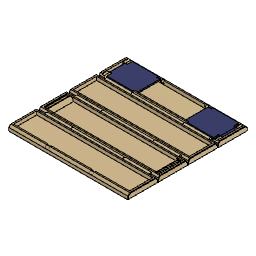
RollupBoard (Autodesk Fusion 360 design; units mm, degrees)
Autodesk Fusion 360 part; units mm, degrees
note: some values were not read from the file. Chosen so that the rebuilt part matches the saved one: a side; which face or edge a step refers to. Set by a fixed rule: which sketch regions a step uses.
sketch "Sketch3" plane through (0, 0, 0) normal (1, 0, 0) x (0, 1, 0)
  line L0 (0.25, 0) -> (45.75, 0)
  line L1 (46, 0) -> (46, 8) construction
  circle A0 centre (46, 5) radius 0.875 construction
  line L2 (38.0198, 12.9802) -> (46, 5) construction
  circle A1 centre (46, 5) radius 1.225
  arc A2 (47.8562, 3.1438) -> (43.9755, 6.6709) centre (46, 5) ccw
  line L3 (47.8562, 3.1438) -> (45.75, 1.0377)
  line L4 (2.9898, 47.3471) -> (2.9889, 8.0542) construction
  line L5 (-5, 5.25) -> (-5, 50.75) construction
  line L6 (43, 8.3536) -> (43, 9.3938) construction
  line L7 (51, 50.75) -> (51, 5.25) construction
  line L8 (24.7755, 27.5722) -> (42.5, 27.5722) construction
  line L9 (42.5, 27.5722) -> (42.5, 9.8477) construction
  line L10 (42.5, 9.8477) -> (24.7755, 9.8477) construction
  line L11 (24.7755, 9.8477) -> (24.7755, 27.5722) construction
  circle A3 centre (13.4891, 17.5722) radius 10 construction
  line L12 (24.7755, 9.8477) -> (42.5, 27.5722) construction
  line L13 (46, 8) -> (42.6464, 8) construction
  line L14 (40.6464, 2.5) -> (40.6464, 8)
  line L15 (3, 10.1318) -> (-3.0001, 10.1756) construction
  line L16 (-3.0001, 45.4688) -> (3, 45.425) construction
  line L17 (-3.0001, 10.1756) -> (-3.0001, 45.4688) construction
  line L18 (48.5, 10.3536) -> (43, 10.3536) construction
  line L19 (49.0395, 45.534) -> (48.5, 10.3536) construction
  line L20 (43.0002, 45.5096) -> (49.0395, 45.534) construction
  circle A4 centre (13.4891, 38.0722) radius 10 construction
  line L21 (-3.0001, 27.8222) -> (-12.3549, 27.8222) construction
  line L22 (5.453, 47.7007) -> (5.4663, 53.6839) construction
  line L23 (5.4663, 53.6839) -> (40.6464, 53.1444) construction
  line L24 (42.6464, 47.6444) -> (41.608, 47.6437) construction
  line L25 (0.25, 55.6444) -> (45.75, 55.6444) construction
  line L26 (40.6464, 53.1444) -> (40.6464, 47.6444) construction
  line L27 (24.7755, 28.0722) -> (42.5, 28.0722) construction
  line L28 (24.7755, 45.7968) -> (24.7755, 28.0722) construction
  line L29 (42.5, 28.0722) -> (42.5, 45.7968) construction
  line L30 (42.5, 45.7968) -> (24.7755, 45.7968) construction
  line L31 (23, 0) -> (23, 6.2006) construction
  line L32 (45.75, 4.8964) -> (42.6464, 8)
  line L33 (45.75, 4.8964) -> (45.75, 0)
  line L34 (44.1438, 3.1438) -> (46.25, 1.0377) construction
  arc A5 (43.9755, 6.6709) -> (44.1438, 3.1438) centre (46, 5) ccw construction
  arc A6 (43.727, 6.9194) -> (43.8964, 2.8964) centre (46, 5) ccw
  line L35 (43.8964, 2.8964) -> (45.75, 1.0427)
  line L36 (2.1036, 2.8964) -> (0.25, 1.0427)
  arc A7 (2.1036, 2.8964) -> (2.273, 6.9194) centre (0, 5) ccw
  line L37 (0.25, 4.8964) -> (3.3536, 8)
  arc A8 (2.0245, 6.6709) -> (-1.8562, 3.1438) centre (0, 5) ccw
  circle A9 centre (0, 5) radius 0.875 construction
  line L38 (-1.8562, 3.1438) -> (0.25, 1.0377)
  line L39 (0.25, 4.8964) -> (0.25, 0)
  line L40 (42.6464, 8) -> (3.3536, 8)
  line L41 (5.3536, 2.5) -> (5.3536, 8)
  line L42 (5.3536, 2.5) -> (40.6464, 2.5)
  circle A10 centre (0, 5) radius 1.225
  circle A11 centre (46, 5) radius 1.115
  point P0 (33.6377, 18.7099)
  dimension "d10" = 46
  dimension "d11" = 1.75
  dimension "d15" = 5
  dimension "d16" = 45
  dimension "d17" = 0.35
  dimension "d18" = 1.75
  dimension "d25" = 17.7245
  dimension "d28" = 20
  dimension "d37" = 20.5
  dimension "d38" = 0.5
  dimension "d39" = 0.5
  dimension "d40" = 10.5
  dimension "d41" = 23
  dimension "d56" = 0.25
  dimension "d57" = 0.25
  dimension "d58" = 45
  dimension "d59" = 0.35
  dimension "d60" = 0.25
  dimension "d61" = 8
  dimension "d62" = 2
  dimension "d63" = 2.5
  dimension "d65" = 0.35
  dimension "d78" = 0.24
  constraint horizontal L0
  constraint vertical L1
  constraint coincident L1 A0.centre
  constraint coincident A0.centre L2.end
  constraint concentric A0 A1
  constraint tangent A2 L3
  constraint coincident L1.start L0
  constraint symmetric L0.end L2 L7.end
  constraint symmetric L13.end L2 L6.start
  constraint symmetric L2 L0.start L7.start
  constraint horizontal L8
  constraint vertical L9
  constraint horizontal L10
  constraint vertical L11
  constraint equal L10 L11
  constraint midpoint L12 P0
  constraint symmetric L2 L14.start L18.start
  constraint symmetric L2 L14.end L18.end
  constraint equal A3 A4
  constraint midpoint L17 L21.start
  constraint perpendicular L17 L21
  constraint symmetric A3.centre A4.centre L21
  constraint symmetric L0.end L21 L25.end
  constraint symmetric L13.end L21 L24.start
  constraint symmetric L0.start L21 L25.start
  constraint symmetric L14.start L21 L23.end
  constraint symmetric L14.end L21 L26.end
  constraint symmetric L8.start L21 L27.start
  constraint symmetric L8.end L21 L27.end
  constraint symmetric L9.end L21 L29.end
  constraint symmetric L10.end L21 L28.start
  constraint perpendicular L0 L31
  constraint coincident L0 L31.start
  constraint parallel L2 L32
  constraint coincident L13.end L32.end
  constraint coincident L32 A2.end
  constraint parallel L1 L33
  constraint coincident L33 L3.end
  constraint symmetric L1 A2.start L34.start
  constraint symmetric L1 L3.end L34.end
  constraint coincident A2.end A5.start
  constraint coincident L32 A6.start
  constraint parallel L34 L35
  constraint coincident A6.end L35.start
  constraint tangent A6 L35
  constraint coincident L33 L35.end
  constraint coincident L0.end L33.end
  constraint coincident origin L0
  constraint vertical L14
  constraint symmetric A0 L31 A9
  constraint symmetric A2.start L31 A8.end
  constraint symmetric A2 L31 A8
  constraint symmetric L32.start L31 L37.start
  constraint symmetric L31 L13.end L37.end
  constraint symmetric L31 A2.end A8.start
  constraint symmetric L31 L0.end L0.start
  constraint symmetric L31 L3.end L38.end
  constraint symmetric L31 A6.start A7.end
  constraint symmetric L31 A6.end L36.start
  constraint symmetric L31 A6 A7
  constraint symmetric L31 L35.end L36.end
  constraint horizontal L40
  constraint coincident L37.end L40.end
  constraint horizontal L13
  constraint coincident L14.end L40
  constraint symmetric L14.start L31 L41.start
  constraint symmetric L14.end L31 L41.end
  constraint concentric A7 A10
  constraint concentric A2 A11
  measures "d10" distance of origin L1.start
  measures "d11" diameter of A0
  measures "d15" distance of L1.start A0.centre
  measures "d16" angle of L1 L2
  measures "d17" distance of A0 A1
  measures "d18" distance of A0 A2
  measures "d25" distance of L8.start L8.end
  measures "d28" diameter of A3
  measures "d37" distance of A3.centre A4.centre
  measures "d38" distance of L8 L27
  measures "d39" distance of L6 L9
  measures "d40" distance of L4 A3.centre
  measures "d41" distance of origin L31.start
  measures "d56" distance of L2 L32
  measures "d57" distance of L1 L33
  measures "d58" angle of L1 L3
  measures "d59" distance of A5 A6
  measures "d60" distance of origin L0.start
  measures "d61" distance of L1.start L1.end
  measures "d62" distance of L13.end L14.end
  measures "d63" distance of L0 L14.start
  measures "d65" distance of A9 A10
  measures "d78" distance of A0 A11
extrude "Extrude2" add sketch "Sketch3" along normal mid plane 184 contours L0 L14 L32 L33 A6 L35 L36 A7 L37 L39 L40 L41 L42 | L36 A7 L37 L39 A10 | A1 L32 L33 A6 L35 | L14 L40 L41 L42 makes body 1
extrude "Extrude3" cut sketch "Sketch3" along normal up to surface (89 mm away) and the other way up to surface (89 mm away) contours L14 L40 L41 L42 bodies 1
extrude "Extrude8" add sketch "Sketch3" along normal blind 40 from surface at 40 contours A1 A2 L3 L32 L33 | A1 L32 L33 A11 | A1 L32 L33 A11 bodies 1
mirror "Mirror3" about plane through (0, 0, 0) normal (1, 0, 0) of "Extrude8"
extrude "Extrude9" cut sketch "Sketch3" along normal up to surface (80 mm away) from surface at -40 contours A1 L32 L33 A6 L35 bodies 1
extrude "Extrude10" add sketch "Sketch3" along normal mid plane 79.3 contours L37 A8 L38 L39 A10 bodies 1
extrude "Extrude11" cut sketch "Sketch3" along normal blind 40.7 from surface at 39.65 contours L36 A7 L37 L39 A10 bodies 1
mirror "Mirror4" about plane through (0, 0, 0) normal (1, 0, 0) of "Extrude11"
copy_body "CopyPasteBodies4" bodies 1 makes body 2
move_body "Move4" bodies 2 to x (1, 0, 0) y (0, 1, 0) z (0, 0, 1) at (0, 46, 0)
extrude "Extrude12" add sketch "Sketch3" along normal mid plane 184 separate body contours L0 L14 L32 L33 A6 L35 L36 A7 L37 L39 L40 L41 L42 | L36 A7 L37 L39 A10 | A1 L32 L33 A6 L35 | L37 L39 A10 | L14 L40 L41 L42 picked at (0.8957, 5.0245) makes body 3
extrude "Extrude13" cut sketch "Sketch3" along normal up to surface (89 mm away) and the other way up to surface (89 mm away) contours L14 L40 L41 L42 bodies 3
extrude "Extrude14" add sketch "Sketch3" along normal blind 40 from surface at 40 contours A1 A2 L3 L32 L33 | A1 L32 L33 A11 | A1 L32 L33 A11 bodies 3
mirror "Mirror5" about plane through (0, 0, 0) normal (1, 0, 0) of "Extrude14"
extrude "Extrude15" cut sketch "Sketch3" along normal up to surface (80 mm away) from surface at -40 contours A1 L32 L33 A6 L35 bodies 3
move_body "Move6" bodies 3 to x (1, 0, 0) y (0, 1, 0) z (0, 0, 1) at (0, -46, 0)
extrude "Extrude16" add sketch "Sketch3" along normal mid plane 184 separate body contours L0 L14 L32 L33 A6 L35 L36 A7 L37 L39 L40 L41 L42 | L36 A7 L37 L39 A10 | A1 L32 L33 A6 L35 | A1 L32 L33 A11 | L32 L33 A11 | L14 L40 L41 L42 picked at (45.6913, 3.8552) picked at (45.2318, 4.6818) makes body 4
extrude "Extrude17" cut sketch "Sketch3" along normal up to surface (89 mm away) and the other way up to surface (89 mm away) contours L14 L40 L41 L42 bodies 4
extrude "Extrude18" add sketch "Sketch3" along normal mid plane 79.3 contours L37 A8 L38 L39 A10 bodies 4
extrude "Extrude19" cut sketch "Sketch3" along normal blind 40.7 from surface at 39.65 contours L36 A7 L37 L39 A10 bodies 4
mirror "Mirror6" about plane through (0, 0, 0) normal (1, 0, 0) of "Extrude19"
move_body "Move7" bodies 4 to x (1, 0, 0) y (0, 1, 0) z (0, 0, 1) at (0, 92, 0)
chamfer "Chamfer1" distance 0.6 angle 45 8 faces at (-92, 16.4512, 2.6667) (92, 16.4512, 2.6667) (-92, -29.5488, 2.6667) (92, -29.5488, 2.6667) (-92, 108.4512, 2.6667) (92, 108.4512, 2.6667) (-92, 62.4512, 2.6667) (92, 62.4512, 2.6667) on bodies 1 2 3 4
sketch "Sketch5" plane through (0, 0, 0) normal (0, 0, 1) x (1, 0, 0)
  circle A0 centre (69, -22) radius 17.5
  circle A1 centre (69, -22) radius 15.5
  circle A2 centre (23, -22) radius 15.5
  circle A3 centre (23, -22) radius 17.5
  circle A4 centre (-23, -22) radius 15.5
  circle A5 centre (-23, -22) radius 17.5
  circle A6 centre (-69, -22) radius 15.5
  circle A7 centre (-69, -22) radius 17.5
  circle A8 centre (69, 24) radius 15.5
  circle A9 centre (69, 24) radius 17.5
  circle A10 centre (23, 24) radius 15.5
  circle A11 centre (23, 24) radius 17.5
  circle A12 centre (-23, 24) radius 15.5
  circle A13 centre (-23, 24) radius 17.5
  circle A14 centre (-69, 24) radius 15.5
  circle A15 centre (-69, 24) radius 17.5
  circle A16 centre (69, 70) radius 15.5
  circle A17 centre (69, 70) radius 17.5
  circle A18 centre (23, 70) radius 15.5
  circle A19 centre (23, 70) radius 17.5
  circle A20 centre (-23, 70) radius 15.5
  circle A21 centre (-23, 70) radius 17.5
  circle A22 centre (-69, 70) radius 15.5
  circle A23 centre (-69, 70) radius 17.5
  circle A24 centre (69, 116) radius 15.5
  circle A25 centre (69, 116) radius 17.5
  circle A26 centre (23, 116) radius 15.5
  circle A27 centre (23, 116) radius 17.5
  circle A28 centre (-23, 116) radius 15.5
  circle A29 centre (-23, 116) radius 17.5
  circle A30 centre (-69, 116) radius 15.5
  circle A31 centre (-69, 116) radius 17.5
  dimension "d146" = 2
  dimension "d147" = 35
  dimension "d148" = 69
  dimension "d149" = 22
  dimension "d152" = -46
  dimension "d153" = 46
  constraint concentric A0 A1
  measures "d146" distance of A0 A1
  measures "d147" diameter of A0
  measures "d148" horizontal distance of A0.centre origin
  measures "d149" vertical distance of A0.centre origin
extrude "Extrude21" cut sketch "Sketch5" along normal blind 0.5 bodies 1 2 3 4
copy_body "Body->Comp1" bodies 1 removing the originals makes body 5 in component "BoardThree"
copy_body "Body->Comp2" bodies 2 removing the originals makes body 6 in component "BoardTwo"
copy_body "Body->Comp3" bodies 3 removing the originals makes body 7 in component "BoardFour"
copy_body "Body->Comp4" bodies 4 removing the originals makes body 8 in component "BoardOne"
sketch "Sketch1" plane through (0, 97.3536, 0) normal (0, 1, 0) x (-1, 0, 0) in component "EndFlap"
  line L0 (-89, 8) -> (-89, 2.5) construction
  line L1 (-89, 2.5) -> (89, 2.5) construction
  line L2 (89, 2.5) -> (89, 8) construction
  line L3 (89, 8) -> (-89, 8) construction
  line L4 (-85, 7.5) -> (-37, 7.5)
  line L5 (-37, 7.5) -> (-37, 5.5)
  line L6 (-37, 5.5) -> (-82.1716, 5.5)
  arc A0 (-85, 7.5) -> (-82.1716, 5.5) centre (-85, 4.5) ccw
  circle A1 centre (-85, 4.5) radius 0.875 construction
  circle A2 centre (-85, 4.5) radius 1.225
  line L7 (91.4, 0) -> (-91.4, 0) construction
  line L8 (-82, 5.5) -> (-82, 7.5)
  dimension "d156" = 2
  dimension "d157" = 1.75
  dimension "d158" = 0.35
  dimension "d159" = 0.5
  dimension "d160" = 4
  dimension "d161" = 3
  dimension "d162" = 1.775
  dimension "d163" = 3.5
  dimension "d164" = 48
  dimension "d192" = 5.5
  constraint parallel L1 L4
  constraint perpendicular L4 L5
  constraint perpendicular L5 L6
  constraint coincident L6.end A0.end
  constraint concentric A0 A1
  constraint concentric A0 A2
  constraint tangent L4 A0
  constraint coincident L6 L8.start
  constraint coincident L4 L8.end
  constraint perpendicular L4 L8
  constraint tangent A0 L8
  measures "d156" distance of L4.end L5.end
  measures "d157" diameter of A1
  measures "d158" distance of A1 A2
  measures "d159" distance of L3 L4
  measures "d160" distance of L0 A0.centre
  measures "d161" radius of A0
  measures "d162" distance of A0 A2
  measures "d163" vertical distance of L0.start A0.centre
  measures "d164" distance of L4.start L4.end
  measures "d192" distance of L0.start L0.end
extrude "Extrude1" add sketch "Sketch1" along normal up to surface (39.2929 mm away) from surface at -2 separate body makes body 9 in component "EndFlap"
extrude "Extrude2'" cut sketch "Sketch1" along normal blind 8 from surface at -2 contours L4 L6 A0 L8 bodies 9 in component "EndFlap"
extrude "Extrude3'" cut sketch "Sketch1" against normal blind 8 from surface at 37.2929 contours L4 L6 A0 L8 bodies 9 in component "EndFlap"
sketch "Sketch2" plane through (0, 0, 7.5) normal (0, 0, 1) x (-1, 0, 0) in component "EndFlap"
  line L0 (-85, -126.6464) -> (-82, -126.6464) construction
  line L1 (-82, -126.6464) -> (-82, -134.6464) construction
  line L2 (-82, -134.6464) -> (-37, -134.6464)
  line L3 (-37, -134.6464) -> (-37, -95.3536)
  line L4 (-37, -95.3536) -> (-82, -95.3536)
  line L5 (-82, -95.3536) -> (-82, -103.3536) construction
  line L6 (-82, -103.3536) -> (-85, -103.3536) construction
  line L7 (-85, -103.3536) -> (-85, -126.6464) construction
  line L8 (-42, -134.6464) -> (-42, -132.1464)
  line L9 (-42, -132.1464) -> (-38, -132.1464)
  line L10 (-38, -132.1464) -> (-37, -131.1464)
  line L11 (-37, -115) -> (-48.9821, -115) construction
  line L12 (-42, -97.8536) -> (-38, -97.8536)
  line L13 (-42, -95.3536) -> (-42, -97.8536)
  line L14 (-38, -97.8536) -> (-37, -98.8536)
  dimension "d199" = 135
  dimension "d200" = 5
  dimension "d201" = 2.5
  dimension "d202" = 1
  constraint coincident L2 L8.start
  constraint perpendicular L2 L8
  constraint perpendicular L8 L9
  constraint coincident L3 L10.end
  constraint midpoint L3 L11.start
  constraint perpendicular L3 L11
  constraint symmetric L8.start L11 L13.start
  constraint symmetric L8.end L11 L12.start
  constraint symmetric L9.end L11 L12.end
  constraint symmetric L10.end L11 L14.end
  measures "d199" angle of L9 L10
  measures "d200" distance of L2.end L8.start
  measures "d201" distance of L8.start L8.end
  measures "d202" distance of L3 L9.end
extrude "Extrude4" cut sketch "Sketch2" against normal through all bodies 9 in component "EndFlap"
sketch "Sketch1 (2)" plane through (0, 97.3536, 0) normal (0, 1, 0) x (-1, 0, 0) in component "BoardOne"
  line L0 (-82, 7.5) -> (-42, 7.5) construction
  line L1 (-38, 7.5) -> (-42, 7.5) construction
  line L2 (-38, 7.5) -> (-38, 5.5) construction
  line L3 (-37, 5.5) -> (-37, 7.5) construction
  arc A0 (-85, 7.5) -> (-82.1716, 5.5) centre (-85, 4.5) ccw construction
  line L4 (-82, 7.5) -> (-85, 7.5) construction
  line L5 (-82, 5.5) -> (-82, 7.5) construction
  line L6 (-42, 5.5) -> (-82, 5.5) construction
  line L7 (-89, 2.5) -> (89, 2.5)
  line L8 (-89, 2.5) -> (-89, 8) construction
  line L9 (-89, 8) -> (89, 8)
  arc A1 (-82, 5.5) -> (-85.8762, 7.5385) centre (-85, 4.5) ccw construction
  line L10 (-82.4183, 5.15) -> (-41.5, 5.15)
  arc A2 (-42, 5.5) -> (-42.3662, 10.1882) centre (-85, 4.5) ccw construction
  line L11 (-41.5, 5.15) -> (-41.5, 8)
  arc A3 (-82.4183, 5.15) -> (-85, 7.1623) centre (-85, 4.5) ccw
  arc A4 (-82, 7.5) -> (-88, 7.5) centre (-85, 4.5) ccw construction
  line L12 (-88, 7.5) -> (-85, 4.5) construction
  line L13 (-85, 4.5) -> (-82, 7.5) construction
  line L14 (-88, 13.4214) -> (-88, 4.5) construction
  line L15 (-88.5, 7.1623) -> (-88.5, 8)
  line L16 (-85, 7.1623) -> (-88.5, 7.1623)
  dimension "d206" = 0.5
  dimension "d207" = 0.35
  dimension "d208" = 0.5
  dimension "d212" = 90
  dimension "d213" = 0.5
  constraint coincident L5.start L6.end
  constraint coincident A0.centre A1.centre
  constraint horizontal L10
  constraint coincident L6.start A2.start
  constraint coincident L9 L11.end
  constraint perpendicular L9 L11
  constraint coincident L0.start L4.start
  constraint perpendicular L9 L14
  constraint coincident A4.end L14
  constraint coincident A0 L14.end
  constraint perpendicular L9 L15
  constraint coincident L9 L15.end
  constraint horizontal L16
  constraint tangent A3 L16
  constraint coincident L15.start L16.end
  measures "d206" horizontal distance of L6.start L10.end
  measures "d207" distance of L6 L10
  measures "d208" distance of A1 A3
  measures "d212" angle of L12 L13
  measures "d213" distance of L14 L15
extrude "Extrude1'" cut sketch "Sketch1 (2)" against normal through all and the other way through all bodies 8 in component "BoardOne"
sketch "Sketch2 (2)" plane through (0, 97.3536, 0) normal (0, 1, 0) x (-1, 0, 0) in component "BoardOne"
  line L0 (-89, 8) -> (-89, 2.5)
  line L1 (-89, 2.5) -> (89, 2.5)
  line L2 (-41.5, 5.15) -> (-82.4183, 5.15)
  arc A0 (-82.4183, 5.15) -> (-85, 7.1623) centre (-85, 4.5) ccw
  line L3 (-85, 7.1623) -> (-88.5, 7.1623)
  circle A1 centre (-85, 4.5) radius 0.875 construction
  circle A2 centre (-85, 4.5) radius 1.115
  line L4 (-82.4183, 5.15) -> (-82.4183, 2.5)
  line L5 (-88.5, 7.1623) -> (-89, 7.1623)
  circle A3 centre (-85, 4.5) radius 3 construction
  arc A4 (-87.6875, 2.5) -> (-82.3125, 2.5) centre (-85, 4.5) ccw
  line L6 (-91.4, 0) -> (91.4, 0) construction
  line L7 (-85, 4.5) -> (-85, 0) construction
  point P0 (-85, 1.15)
  dimension "d216" = 1.75
  dimension "d217" = 0.24
  dimension "d245" = 6
  dimension "d246" = 0.35
  dimension "d250" = 1.15
  constraint concentric A0 A1
  constraint concentric A1 A2
  constraint coincident L2.end A0.start
  constraint coincident L1 L4.end
  constraint perpendicular L1 L4
  constraint coincident L3.end L5.start
  constraint coincident L0 L5.end
  constraint perpendicular L0 L5
  constraint concentric A1 A3
  constraint coincident L1 A4.end
  constraint coincident L1 A4.start
  constraint coincident A0.centre A1.centre
  constraint coincident L6 L7.end
  constraint perpendicular L6 L7
  constraint midpoint A4 P0
  measures "d216" diameter of A1
  measures "d217" distance of A1 A2
  measures "d245" diameter of A3
  measures "d246" distance of A3 A4
  measures "d250" distance of L7.end P0
extrude "Extrude3''" add sketch "Sketch2 (2)" along normal blind 5.65 contours L0 L1 A0 L3 L4 L5 bodies 8 in component "BoardOne"
extrude "Extrude4'" add sketch "Sketch2 (2)" against normal blind 5.65 from surface at 35.2929 contours L0 L1 A0 L3 L4 L5 bodies 8 in component "BoardOne"
extrude "Extrude5" cut sketch "Sketch2 (2)" along normal through all and the other way through all contours A2 bodies 8 in component "BoardOne"
extrude "Extrude6" cut sketch "Sketch2 (2)" along normal up to surface (23.9929 mm away) from surface at 5.65 contours L1 A4 bodies 8 in component "BoardOne"
mirror "Mirror1" about plane through (0, 0, 0) normal (1, 0, 0) of "Extrude1'", "Extrude3''", "Extrude4'", "Extrude5", "Extrude6" in component "BoardOne"
mirror "MirrorComponent1" about plane through (0, 0, 0) normal (0, 0, 1) of bodies 9 makes body 10 in component "EndFlap(Mirror)"
sketch "Sketch2 (3)" plane through (0, 5.3536, 0) normal (0, 1, 0) x (-1, 0, 0) in component "BoardThree"
  line L0 (-88, 13.4214) -> (-88, 4.5) construction
  line L1 (-89, 8) -> (-89, 2.5)
  line L2 (-89, 2.5) -> (89, 2.5)
  line L3 (89, 8) -> (-89, 8)
  line L4 (-86, 2.5) -> (-86, 10.6426) construction
  line L5 (-88, 4.5) -> (-88, 2.5) construction
  line L6 (-88.35, 2.5) -> (-88.35, 6.5)
  line L7 (-85.65, 2.5) -> (-85.65, 6.5)
  line L8 (-88.35, 6.5) -> (-89, 7.15)
  line L9 (-85.65, 6.5) -> (-84.65, 7.5)
  line L10 (-84.65, 7.5) -> (-83.65, 7.5)
  arc A0 (-78.65, 2.5) -> (-83.65, 7.5) centre (-83.65, 2.5) ccw
  dimension "d232" = 2
  dimension "d233" = 0.35
  dimension "d234" = 0.35
  dimension "d235" = 4
  dimension "d236" = 135
  dimension "d237" = 135
  dimension "d239" = 1
  dimension "d244" = 1
  constraint coincident L0.end L5.start
  constraint coincident L2 L5.end
  constraint perpendicular L2 L5
  constraint coincident L2 L4.start
  constraint vertical L4
  constraint coincident L2 L6.start
  constraint perpendicular L2 L6
  constraint coincident L2 L7.start
  constraint perpendicular L2 L7
  constraint coincident L1 L8.end
  constraint horizontal L6.end L7.end
  constraint horizontal L10
  constraint coincident L2 A0.start
  constraint tangent L10 A0
  constraint coincident L2 A0.centre
  measures "d232" distance of L4.start L5.end
  measures "d233" distance of L5.end L6.start
  measures "d234" distance of L4 L7
  measures "d235" distance of L6.start L6.end
  measures "d236" angle of L6 L8
  measures "d237" angle of L7 L9
  measures "d239" distance of L9.end L10.end
  measures "d244" vertical distance of L7.end L9.end
extrude "Extrude1''" add sketch "Sketch2 (3)" along normal up to surface (35.2929 mm away) bodies 5 in component "BoardThree"
mirror "Mirror1'" about plane through (0, 0, 0) normal (1, 0, 0) of "Extrude1''" in component "BoardThree"
sketch "Sketch3 (2)" plane through (0, 71.3232, 71.3232) normal (0, 0.707107, 0.707107) x (-1, 0, 0) in component "BoardOne"
  line L0 (-41.5, -89.5526) -> (-41.5, -93.5831) construction
  line L1 (-41.5, -93.5831) -> (-82.4183, -93.5831) construction
  circle A0 centre (-34, -91.3383) radius 2.35 construction
  line L2 (41.5, -88.1383) -> (-41.5, -88.1383)
  line L3 (82.4183, -92.0274) -> (-82.4183, -92.0274) construction
  line L4 (-34, -88.1383) -> (-34, -93.9416) construction
  line L5 (-36.59, -88.1383) -> (-36.59, -91.3383)
  arc A1 (-36.59, -91.3383) -> (-31.41, -91.3383) centre (-34, -91.3383) ccw
  line L6 (-31.41, -91.3383) -> (-31.41, -88.1383)
  line L7 (-83.9579, -93.9416) -> (83.9579, -93.9416) construction
  line L8 (0, -88.1383) -> (0, -71.6518) construction
  line L9 (-34, -76.794) -> (-34, -88.1383) construction
  line L10 (82.4183, -93.5831) -> (41.5, -93.5831)
  line L11 (41.5, -93.5831) -> (41.5, -89.5526)
  line L12 (41.5, -89.5526) -> (-41.5, -89.5526) construction
  line L13 (36.59, -88.1383) -> (36.59, -91.3383)
  arc A2 (31.41, -91.3383) -> (36.59, -91.3383) centre (34, -91.3383) ccw
  line L14 (31.41, -91.3383) -> (31.41, -88.1383)
  dimension "d251" = 4.7
  dimension "d260" = 0.24
  dimension "d297" = 34
  dimension "d301" = 3.2
  constraint coincident A0.centre L4
  constraint perpendicular L2 L5
  constraint tangent L5 A1
  constraint perpendicular L2 L6
  constraint tangent A1 L6
  constraint coincident A0.centre A1.centre
  constraint coincident L4.end L7
  constraint coincident L2 L5.start
  constraint coincident L2 L6.end
  constraint vertical L4
  constraint coincident L2 L4.start
  constraint vertical L9
  constraint midpoint L2 L8.start
  constraint symmetric L5.start L8 L13.start
  constraint symmetric L5.end L8 L13.end
  constraint symmetric A1.end L8 A2.start
  constraint symmetric A1 L8 A2
  constraint symmetric L6.end L8 L14.end
  measures "d251" diameter of A0
  measures "d260" distance of A0 A1
  measures "d297" distance of L8 L9
  measures "d301" distance of A0.centre L4.start
extrude "Extrude8'" cut sketch "Sketch3 (2)" against normal blind 3.655 from surface at -0.6 bodies 8 in component "BoardOne"
sketch "Sketch1 (3)" plane through (0, -25.3232, 25.3232) normal (0, -0.707107, 0.707107) x (1, 0, 0) in component "BoardFour"
  line L0 (91.4, -28.8878) -> (91.4, -24.4987)
  line L1 (91.4, -24.4987) -> (-91.4, -24.4987) construction
  line L2 (-91.4, -24.4987) -> (-91.4, -28.8878)
  line L3 (-91.4, -28.8878) -> (91.4, -28.8878) construction
  line L4 (-36.59, -23.0845) -> (-36.59, -26.2845)
  line L5 (-31.41, -26.2845) -> (-31.41, -23.0845)
  circle A0 centre (-34, -26.2845) radius 2.35 construction
  arc A1 (-36.59, -26.2845) -> (-31.41, -26.2845) centre (-34, -26.2845) ccw
  line L6 (-34, -24.4987) -> (-34, -28.8878) construction
  line L7 (89, -23.0845) -> (-89, -23.0845)
  line L8 (0, 0) -> (0, -23.0845) construction
  arc A2 (31.41, -26.2845) -> (36.59, -26.2845) centre (34, -26.2845) ccw
  line L9 (31.41, -26.2845) -> (31.41, -23.0845)
  line L10 (36.59, -23.0845) -> (36.59, -26.2845)
  dimension "d286" = 4.7
  dimension "d288" = 0.24
  dimension "d299" = 34
  dimension "d300" = 3.2
  constraint coincident A0.centre L6
  constraint tangent L4 A1
  constraint tangent L5 A1
  constraint coincident A0.centre A1.centre
  constraint vertical L6
  constraint vertical L5
  constraint vertical L4
  constraint coincident L5.end L7
  constraint coincident L4.start L7
  constraint coincident L8.start origin
  constraint midpoint L7 L8.end
  constraint symmetric L4.start L8 L10.start
  constraint symmetric L4.end L8 A2.end
  constraint symmetric L5.start L8 A2.start
  constraint symmetric L5.end L8 L9.end
  constraint symmetric A1 L8 A2
  constraint coincident L1 L6.start
  constraint coincident L3 L6.end
  measures "d286" diameter of A0
  measures "d288" distance of A0 A1
  measures "d299" distance of L6 L8.end
  measures "d300" distance of A0.centre L7
extrude "Extrude1'''" cut sketch "Sketch1 (3)" against normal blind 3.655 from surface at -0.6 bodies 7 in component "BoardFour"
other "ClearanceTest" in component "BoardFour"
component "BoardThree" placed x (1, 0, 0) y (0, -1, -0.000243) z (0, 0.000243, -1) at (0, 137.9877, 56.0112)
component "BoardTwo" placed x (1, 0, 0) y (0, 0.000242, -1) z (0, 1, 0.000242) at (0, 86.9778, 96.9988)
component "BoardFour" placed x (1, 0, 0) y (0, -0.000886, 1) z (0, -1, -0.000886) at (0, 142.9889, 51.0156)
component "BoardOne" placed x (1, 0, 0) y (0, 1, 0) z (0, 0, 1) at (0, 0, 0)
component "EndFlap" placed x (0, 0, -1) y (0, 1, 0) z (1, 0, 0) at (80.5, 0, 89.5)
component "EndFlap(Mirror)" placed x (0, 0, -1) y (0, 1, 0) z (1, 0, 0) at (-80.5, 0, 89.5)
equation "fit_clr = 0.24 mm"
equation "run_clr = 0.35 mm"
equation "fold_gap = 0.25 mm"
equation "d10 = ( 2.3 * Diam ) * 1 mm"
equation "d17 = run_clr"
equation "d25 = ( Side * 1 ) * 1 mm"
equation "Diam = 20"
equation "Side = sqrt(PI * ( ( Diam / 2 ) ^ 2 ))" comment "square pieces same area as round"
equation "d28 = ( Diam * 1 ) * 1 mm"
equation "d29 = ( Diam / 2 ) * 1 mm + 0.5 mm"
equation "d30 = ( Side / 2 ) * 1 mm + 0.5 mm"
equation "d37 = ( ( Diam + 0.5 ) * 1 ) * 1 mm"
equation "d40 = ( Diam / 2 ) * 1 mm + 0.5 mm"
equation "d41 = d10 / 2"
equation "d42 = ( Diam * 9.2 ) * 1 mm"
equation "d56 = fold_gap"
equation "d57 = fold_gap"
equation "d59 = run_clr"
equation "d60 = fold_gap"
equation "d65 = run_clr"
equation "d78 = fit_clr"
equation "d96 = 80 mm - 2 * run_clr"
equation "d99 = 40 mm + 2 * run_clr"
equation "d111 = ( 9.2 * Diam ) * 1 mm"
equation "d125 = ( 9.2 * Diam ) * 1 mm"
equation "d131 = 80 mm - 2 * run_clr"
equation "d134 = 40 mm + 2 * run_clr"
equation "d147 = ( Diam * 1.75 ) * 1 mm"
equation "d148 = ( Diam * 3.45 ) * 1 mm"
equation "d149 = ( 1.1 * Diam ) * 1 mm"
equation "d152 = ( -2.3 * Diam ) * 1 mm"
equation "d153 = ( 2.3 * Diam ) * 1 mm"
equation "d158 = run_clr"
equation "d207 = run_clr"
equation "d217 = fit_clr"
equation "d218 = 6 mm - run_clr"
equation "d221 = -6 mm + run_clr"
equation "d233 = run_clr"
equation "d234 = run_clr"
equation "d246 = run_clr"
equation "d257 = -0'- 1/8\" - 2 * fit_clr"
equation "d260 = fit_clr"
equation "d288 = fit_clr"
equation "d290 = -0'- 1/8\" - 2 * fit_clr"
named bodies: "Middle", "Middle2", "Start", "End"
